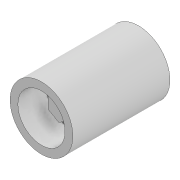
# Autodesk Inventor part: driver gear adapter
Saved by Autodesk Inventor 2022 (Build 260153000, 153)
## iProperties
Created: 2024-05-31
Part Number: driver gear adapter
Material: Generic
Document SubType Name: Modeling
Designer: david
Density: 1 g/cm^3
Appearance: Default
Author: david
Autodesk Inventor part; units mm, degrees
ref_plane "YZ Plane" through (0, 0, 0) normal (1, 0, 0) x (0, 1, 0)
ref_plane "XZ Plane" through (0, 0, 0) normal (0, 1, 0) x (-1, 0, 0)
ref_plane "XY Plane" through (0, 0, 0) normal (0, 0, 1) x (1, 0, 0)
sketch "Sketch1" plane through (0, 0, 0) normal (0, 0, 1) x (1, 0, 0)
  circle A0 centre (0, 0) radius 5.5
  dimension "d1" = 11
  constraints: 1 centre point, 1 coincident
  measures "d1" diameter of A0
extrude "Extrusion1" add sketch "Sketch1" along normal blind 10 and the other way blind 7
sketch "Sketch2" plane through (0, 0, 10) normal (0, 0, 1) x (1, 0, 0)
  circle A0 centre (0, 0) radius 5.5 projected
  constraints: 1 coincident
hole "Hole1" at (0, 0, 10) direction (0, 0, -1) diameter 8 depth 5
sketch "Sketch3" plane through (0, 0, 5) normal (0, 0, 1) x (1, 0, 0)
  circle A0 centre (0, 0) radius 5.5 projected
  constraints: 1 coincident
hole "Hole2" at (0, 0, 5) direction (0, 0, -1) diameter 6.3 depth 4
sketch "Sketch4" plane through (0, 0, 1) normal (0, 0, 1) x (1, 0, 0)
  line L0 (-2, 1.1547) -> (0, 2.3094)
  line L1 (0, 2.3094) -> (2, 1.1547)
  line L2 (2, 1.1547) -> (2, -1.1547)
  line L3 (2, -1.1547) -> (0, -2.3094)
  line L4 (0, -2.3094) -> (-2, -1.1547)
  line L5 (-2, -1.1547) -> (-2, 1.1547)
  point P0 (0, 0)
  point P1 (0, 0)
  dimension "d20" = 4
  constraints: 12 end point, 1 coincident, 1 vertical, 13 other
  measures "d20" distance between parallel lines of L5 L2
extrude "Extrusion2" add sketch "Sketch4" along normal blind 6
sketch "Sketch5" plane through (0, 0, -7) normal (0, 0, -1) x (-1, 0, 0)
  arc A0 (-1.8875, 2) -> (-1.8875, -2) centre (0, 0) ccw construction
  line L0 (-1.8875, -2) -> (1.8875, -2) construction
  line L1 (1.8875, -2) -> (1.8875, 2)
  line L2 (1.8875, 2) -> (-1.8875, 2) construction
  line L3 (-1.8875, 2) -> (-1.8875, -2)
  line L4 (-1.8875, -2) -> (1.8875, 2) construction
  line L5 (1.8875, -2) -> (0, 0) construction
  arc A1 (1.8875, 2) -> (-1.8875, 2) centre (0, 0) ccw
  arc A2 (1.8875, -2) -> (1.8875, 2) centre (0, 0) ccw construction
  arc A3 (-1.8875, -2) -> (1.8875, -2) centre (0, 0) ccw
  line L6 (0, 0) -> (-1.8875, 2) construction
  dimension "d23" = 5.5
  dimension "d24" = 4
  constraints: 14 end point, 8 point on circle, 4 centre point, 2 coincident, 2 midpoint, 2 parallel, 1 horizontal, 1 perpendicular
  measures "d23" diameter of A0
  measures "d24" distance of L1.end L0.end
extrude "Extrusion3" cut sketch "Sketch5" against normal blind 6
thicken "Thicken1" operation add thickness 0.15 both sides no extend neighbours yes toward (-1, 0, 0) faces at (2, -0.3849, 3) (1.3333, 1.5396, 3) (-0.6667, 1.9245, 3) (-2, 0.3849, 3) (-1.3333, -1.5396, 3) (0.6667, -1.9245, 3)
thicken "Thicken2" operation add thickness 0.15 both sides no extend neighbours yes toward (0.1604113, -0.9870503, 0) faces at (0.5053, -3.1092, 3.6667)
thicken "Thicken3" operation add thickness 0.13 both sides no extend neighbours yes toward (0.1604113, -0.9870503, 0) faces at (0.6416, -3.9482, 8.3333)
thicken "Thicken4" operation add thickness 0.13 both sides no extend neighbours yes toward (-1, 0, 0) faces at (-1.8875, 0.6667, -3) (-0.6861, -2.663, -3) (1.5807, 2.2503, -3) (1.8875, 0.6667, -5)
body "Solid1"
